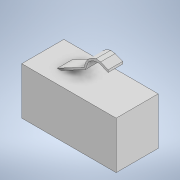
# Autodesk Inventor part: WK330
Saved by Autodesk Inventor 2021 (Build 250183000, 183)
## iProperties
Created: 2021-01-13
Part Number: WK330
Material: Generic
Document SubType Name: Modeling
Designer: awitc
Density: 1 g/cm^3
Appearance: Default
Author: awitc
Autodesk Inventor part; units mm, degrees
ref_plane "YZ Plane" through (0, 0, 0) normal (1, 0, 0) x (0, 1, 0)
ref_plane "XZ Plane" through (0, 0, 0) normal (0, 1, 0) x (-1, 0, 0)
ref_plane "XY Plane" through (0, 0, 0) normal (0, 0, 1) x (1, 0, 0)
sketch "Sketch1" plane through (0, 0, 0) normal (0, 1, 0) x (-1, 0, 0)
  line L0 (13, -10) -> (0, -10)
  line L1 (0, -10) -> (13, -10)
  line L2 (13, -10) -> (13, -4.2)
  line L3 (13, -4.2) -> (0, -4.2)
  line L4 (0, -4.2) -> (0, -10)
  dimension "d0" = 13
  dimension "d4" = 5.8
  constraints: 10 end point, 2 parallel, 1 horizontal, 1 perpendicular
  measures "d0" distance of L0.start L0.end
  measures "d4" distance of L2.end L1.end
extrude "Extrusion1" add sketch "Sketch1" along normal blind 6.5
sketch "Sketch2" plane through (0, 6.5, 0) normal (0, 1, 0) x (1, 0, 0)
  line L0 (0, 4.2) -> (0, 10) projected
  line L1 (0, 0) -> (0, 4.2)
  line L2 (0, 4.2) -> (0, 10)
  line L3 (0, 4.2) -> (0, 10) projected
  line L4 (0, 7.1) -> (-3, 7.1)
  line L5 (-3, 7.1) -> (-3, 8.1)
  line L6 (-3, 8.1) -> (-3, 6.1)
  line L7 (-3, 8.1) -> (-10, 8.1)
  line L8 (-10, 8.1) -> (-10, 6.1)
  line L9 (-10, 6.1) -> (-3, 6.1)
  line L10 (-3, 6.1) -> (-3, 8.1)
  dimension "d5" = 3
  dimension "d6" = 1
  dimension "d7" = 2
  dimension "d8" = 7
  constraints: 18 end point, 3 equal length, 2 horizontal, 2 perpendicular, 1 midpoint, 1 point on line, 1 vertical
  measures "d5" distance of L4.start L4.end
  measures "d6" distance of L4.end L5.end
  measures "d7" distance of L5.end L6.end
  measures "d8" distance of L9.end L8.end
extrude "Extrusion2" add sketch "Sketch2" along normal blind 6
sketch "Sketch3" plane through (-10, 6.5, -6.1) normal (0, 0, 1) x (1, 0, 0)
  line L0 (7, 0) -> (0, 0) projected
  line L1 (0, 0) -> (3.7445, 1.9981)
  line L2 (3.7445, 1.9981) -> (3.8617, 1.7785)
  line L3 (3.8617, 1.7785) -> (0.5288, 0)
  arc A0 (5.3386, 3.8121) -> (3.7445, 1.9981) centre (5.7324, 1.8586) ccw
  arc A1 (5.8481, 3.4507) -> (4.2692, 2.8715) centre (5.5714, 1.7635) ccw
  line L4 (5.9577, 3.7284) -> (7.4262, 3.1492)
  line L5 (7.4262, 3.1492) -> (7.3166, 2.8715)
  line L6 (7.3166, 2.8715) -> (5.8481, 3.4507)
  line L7 (5.3386, 3.8121) -> (5.9577, 3.7284)
  line L8 (3.8617, 1.7785) -> (4.2692, 2.8715)
  line L9 (0.5288, 0) -> (0, 0)
  line L10 (7, 6) -> (0, 6) projected
  line L11 (0, 6) -> (7, 6)
  line L12 (7, 6) -> (7, 0)
  line L13 (7, 0) -> (0, 0)
  line L14 (0, 0) -> (0, 6)
  point P0 (10, -6.5)
  point P1 (7, 2.9964)
  point P2 (7, 3.3173)
  constraints: 26 end point, 5 perpendicular, 4 point on circle, 2 centre point, 2 parallel, 1 collinear, 1 horizontal, 1 point on line
extrude "Extrusion3" cut sketch "Sketch3" against normal blind 6 contours L0 L3 L8 A1 L6 L12 | L14 L10 L12 L4 L7 A0 L1
body "Solid1"
